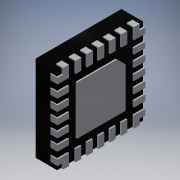
# Autodesk Inventor part: MAX32664GTGA+
Saved by Autodesk Inventor 2018.3 (Build 223284000, 284)
## iProperties
Created: 2021-06-02
Part Number: MAX32664GTGA+
Material: Genérico
Document SubType Name: Modeling
Designer: laguerre
Density: 8.47 g/cm^3
Appearance: Negro
Author: laguerre
Autodesk Inventor part; units mm, degrees
note: some values were not read from the file. Chosen so that the rebuilt part matches the saved one: direction of "Repujado1".
ref_plane "YZ Plane" through (0, 0, 0) normal (1, 0, 0) x (0, 1, 0)
ref_plane "XZ Plane" through (0, 0, 0) normal (0, 1, 0) x (-1, 0, 0)
ref_plane "XY Plane" through (0, 0, 0) normal (0, 0, 1) x (1, 0, 0)
sketch "Boceto39" plane through (0, 0, 0) normal (0, 0, 1) x (1, 0, 0)
  line L0 (-1.5, 1.5) -> (1.5, 1.5)
  line L1 (1.5, 1.5) -> (1.5, -1.5)
  line L2 (1.5, -1.5) -> (-1.5, -1.5)
  line L3 (-1.5, -1.5) -> (-1.5, 1.5)
  point P0 (0, 0)
  point P1 (0, 1.5)
  point P2 (-1.5, 0)
  dimension "d373" = 3
  dimension "d374" = 3
  constraints: 8 end point, 2 midpoint, 2 parallel, 1 horizontal, 1 horizontal alignment, 1 perpendicular, 1 vertical alignment
  measures "d373" distance of L0.start L0.end
  measures "d374" distance of L2.end L0.start
extrude "Extrusión13" add sketch "Boceto39" along normal blind 0.75
sketch "Boceto40" plane through (0, 0, 0.75) normal (0, 0, 1) x (1, 0, 0)
  circle A0 centre (-1.1, 1.1) radius 0.15
  line L0 (-1.5, 1.5) -> (-1.5, -1.5) projected
  line L1 (1.5, 1.5) -> (-1.5, 1.5) projected
  point P0 (0, 0)
  dimension "d377" = 0.4
  dimension "d378" = 0.4
  dimension "d379" = 0.3
  constraints: 1 centre point
  measures "d377" distance from line of L0 A0.centre
  measures "d378" distance from line of A0.centre L1
  measures "d379" diameter of A0
emboss "Repujado1" sketch "Boceto40" operation cut depth 0.001 direction (0, 0, -1)
sketch "Boceto41" plane through (0, 0, 0) normal (0, 0, -1) x (-1, 0, 0)
  line L0 (-0.1, 1.535) -> (0.1, 1.535)
  line L1 (0.1, 1.535) -> (0.1, 1.135)
  line L2 (0.1, 1.135) -> (-0.1, 1.135)
  line L3 (-0.1, 1.135) -> (-0.1, 1.535)
  line L4 (0.3, 1.535) -> (0.5, 1.535)
  line L5 (0.5, 1.535) -> (0.5, 1.135)
  line L6 (0.5, 1.135) -> (0.3, 1.135)
  line L7 (0.3, 1.135) -> (0.3, 1.535)
  line L8 (0.7, 1.535) -> (0.9, 1.535)
  line L9 (0.9, 1.535) -> (0.9, 1.135)
  line L10 (0.9, 1.135) -> (0.7, 1.135)
  line L11 (0.7, 1.135) -> (0.7, 1.535)
  line L12 (-0.5, 1.535) -> (-0.3, 1.535)
  line L13 (-0.3, 1.535) -> (-0.3, 1.135)
  line L14 (-0.3, 1.135) -> (-0.5, 1.135)
  line L15 (-0.5, 1.135) -> (-0.5, 1.535)
  line L16 (-0.9, 1.535) -> (-0.7, 1.535)
  line L17 (-0.7, 1.535) -> (-0.7, 1.135)
  line L18 (-0.7, 1.135) -> (-0.9, 1.135)
  line L19 (-0.9, 1.135) -> (-0.9, 1.535)
  line L20 (-0.1, -1.135) -> (0.1, -1.135)
  line L21 (0.1, -1.135) -> (0.1, -1.535)
  line L22 (0.1, -1.535) -> (-0.1, -1.535)
  line L23 (-0.1, -1.535) -> (-0.1, -1.135)
  line L24 (0.3, -1.135) -> (0.5, -1.135)
  line L25 (0.5, -1.135) -> (0.5, -1.535)
  line L26 (0.5, -1.535) -> (0.3, -1.535)
  line L27 (0.3, -1.535) -> (0.3, -1.135)
  line L28 (0.7, -1.135) -> (0.9, -1.135)
  line L29 (0.9, -1.135) -> (0.9, -1.535)
  line L30 (0.9, -1.535) -> (0.7, -1.535)
  line L31 (0.7, -1.535) -> (0.7, -1.135)
  line L32 (-0.5, -1.135) -> (-0.3, -1.135)
  line L33 (-0.3, -1.135) -> (-0.3, -1.535)
  line L34 (-0.3, -1.535) -> (-0.5, -1.535)
  line L35 (-0.5, -1.535) -> (-0.5, -1.135)
  line L36 (-0.9, -1.135) -> (-0.7, -1.135)
  line L37 (-0.7, -1.135) -> (-0.7, -1.535)
  line L38 (-0.7, -1.535) -> (-0.9, -1.535)
  line L39 (-0.9, -1.535) -> (-0.9, -1.135)
  line L40 (1.135, 0.9) -> (1.535, 0.9)
  line L41 (1.535, 0.9) -> (1.535, 0.7)
  line L42 (1.535, 0.7) -> (1.135, 0.7)
  line L43 (1.135, 0.7) -> (1.135, 0.9)
  line L44 (1.135, 0.5) -> (1.535, 0.5)
  line L45 (1.535, 0.5) -> (1.535, 0.3)
  line L46 (1.535, 0.3) -> (1.135, 0.3)
  line L47 (1.135, 0.3) -> (1.135, 0.5)
  line L48 (1.535, 0.1) -> (1.135, 0.1)
  line L49 (1.135, 0.1) -> (1.135, -0.1)
  line L50 (1.135, -0.1) -> (1.535, -0.1)
  line L51 (1.535, -0.1) -> (1.535, 0.1)
  line L52 (1.135, -0.3) -> (1.535, -0.3)
  line L53 (1.535, -0.3) -> (1.535, -0.5)
  line L54 (1.535, -0.5) -> (1.135, -0.5)
  line L55 (1.135, -0.5) -> (1.135, -0.3)
  line L56 (1.535, -0.7) -> (1.135, -0.7)
  line L57 (1.135, -0.7) -> (1.135, -0.9)
  line L58 (1.135, -0.9) -> (1.535, -0.9)
  line L59 (1.535, -0.9) -> (1.535, -0.7)
  line L60 (-1.535, 0.9) -> (-1.135, 0.9)
  line L61 (-1.135, 0.9) -> (-1.135, 0.7)
  line L62 (-1.135, 0.7) -> (-1.535, 0.7)
  line L63 (-1.535, 0.7) -> (-1.535, 0.9)
  line L64 (-1.535, 0.5) -> (-1.135, 0.5)
  line L65 (-1.135, 0.5) -> (-1.135, 0.3)
  line L66 (-1.135, 0.3) -> (-1.535, 0.3)
  line L67 (-1.535, 0.3) -> (-1.535, 0.5)
  line L68 (-1.135, 0.1) -> (-1.535, 0.1)
  line L69 (-1.535, 0.1) -> (-1.535, -0.1)
  line L70 (-1.535, -0.1) -> (-1.135, -0.1)
  line L71 (-1.135, -0.1) -> (-1.135, 0.1)
  line L72 (-1.535, -0.3) -> (-1.135, -0.3)
  line L73 (-1.135, -0.3) -> (-1.135, -0.5)
  line L74 (-1.135, -0.5) -> (-1.535, -0.5)
  line L75 (-1.535, -0.5) -> (-1.535, -0.3)
  line L76 (-1.135, -0.7) -> (-1.535, -0.7)
  line L77 (-1.535, -0.7) -> (-1.535, -0.9)
  line L78 (-1.535, -0.9) -> (-1.135, -0.9)
  line L79 (-1.135, -0.9) -> (-1.135, -0.7)
  line L80 (1.5, 1.5) -> (-1.5, 1.5) projected
  line L81 (1.5, -1.5) -> (1.5, 1.5) projected
  line L82 (-1.5, 1.5) -> (-1.5, -1.5) projected
  line L83 (-1.5, -1.5) -> (1.5, -1.5) projected
  line L84 (1.135, 1.535) -> (1.135, 1.135)
  line L85 (1.135, 1.135) -> (1.535, 1.135)
  line L86 (1.535, 1.135) -> (1.535, 1.335)
  line L87 (1.535, 1.335) -> (1.335, 1.335)
  line L88 (1.335, 1.335) -> (1.335, 1.535)
  line L89 (-1.5, 1.5) -> (1.5, 1.5) projected
  line L90 (1.335, 1.535) -> (1.135, 1.535)
  line L91 (-1.135, 1.535) -> (-1.135, 1.135)
  line L92 (-1.135, 1.135) -> (-1.535, 1.135)
  line L93 (-1.535, 1.135) -> (-1.535, 1.335)
  line L94 (-1.535, 1.335) -> (-1.335, 1.335)
  line L95 (-1.335, 1.335) -> (-1.335, 1.535)
  line L96 (-1.335, 1.535) -> (-1.135, 1.535)
  line L97 (1.135, -1.135) -> (1.135, -1.535)
  line L98 (1.135, -1.535) -> (1.335, -1.535)
  line L99 (1.335, -1.535) -> (1.335, -1.335)
  line L100 (1.335, -1.335) -> (1.535, -1.335)
  line L101 (1.535, -1.335) -> (1.535, -1.135)
  line L102 (1.535, -1.135) -> (1.135, -1.135)
  line L103 (-1.535, -1.135) -> (-1.135, -1.135)
  line L104 (-1.135, -1.135) -> (-1.135, -1.535)
  line L105 (-1.135, -1.535) -> (-1.335, -1.535)
  line L106 (-1.335, -1.535) -> (-1.335, -1.335)
  line L107 (-1.335, -1.335) -> (-1.535, -1.335)
  line L108 (-1.535, -1.335) -> (-1.535, -1.135)
  line L109 (-0.85, 0.85) -> (0.55, 0.85)
  line L110 (0.85, 0.55) -> (0.85, -0.85)
  line L111 (0.85, -0.85) -> (-0.85, -0.85)
  line L112 (-0.85, -0.85) -> (-0.85, 0.85)
  line L113 (0.55, 0.85) -> (0.85, 0.55)
  point P0 (0, 0)
  point P1 (0, -1.135)
  point P2 (0, 1.135)
  point P3 (0.4, -1.135)
  point P4 (0.4, 1.135)
  point P5 (0.8, 1.135)
  point P6 (0.8, -1.135)
  point P7 (-0.4, -1.135)
  point P8 (-0.4, 1.135)
  point P9 (-0.8, -1.135)
  point P10 (-0.8, 1.135)
  point P11 (1.135, 0)
  point P12 (-1.535, 0)
  point P13 (-1.135, 0.8)
  point P14 (1.135, 0.8)
  point P15 (1.135, 0.4)
  point P16 (-1.135, 0.4)
  point P17 (-1.135, 0)
  point P18 (-1.135, -0.4)
  point P19 (1.135, -0.4)
  point P20 (1.135, -0.8)
  point P21 (-1.135, -0.8)
  point P22 (0.85, 0.85)
  point P23 (-0.85, 0)
  point P24 (0, -0.85)
  dimension "d382" = 0.2
  dimension "d384" = 0.4
  dimension "d385" = 0.2
  dimension "d386" = 0.4
  dimension "d387" = 0.4
  dimension "d388" = 0.4
  dimension "d389" = 0.4
  dimension "d390" = 0.4
  dimension "d391" = 0.4
  dimension "d392" = 0.4
  dimension "d393" = 0.4
  dimension "d394" = 0.4
  dimension "d396" = 0.035
  dimension "d397" = 0.035
  dimension "d398" = 0.035
  dimension "d399" = 0.035
  dimension "d400" = 0.3
  dimension "d401" = 0.3
  dimension "d402" = 1.7
  constraints: 218 end point, 42 parallel, 39 equal length, 39 perpendicular, 23 midpoint, 22 horizontal, 20 collinear, 20 point on line, 7 horizontal alignment, 7 vertical alignment, 3 vertical
  measures "d382" distance of L0.start L0.end
  measures "d384" distance of L2.end L0.start
  measures "d385" distance of L20.start L20.end
  measures "d386" distance of L22.end L20.start
  measures "d387" distance of point (0.4, -1.135) point (0, -1.135)
  measures "d388" distance of point (0.8, -1.135) point (0.4, -1.135)
  measures "d389" distance of point (0, -1.135) point (-0.4, -1.135)
  measures "d390" distance of point (-0.4, -1.135) point (-0.8, -1.135)
  measures "d391" distance of point (-1.135, 0.8) point (-1.135, 0.4)
  measures "d392" distance of point (-1.135, 0.4) point (-1.135, 0)
  measures "d393" distance of point (-1.135, -0.4) point (-1.135, 0)
  measures "d394" distance of point (-1.135, -0.4) point (-1.135, -0.8)
  measures "d396" distance between parallel lines of L8 L80
  measures "d397" distance between parallel lines of L81 L41
  measures "d398" distance between parallel lines of L82 L63
  measures "d399" distance between parallel lines of L83 L30
  measures "d400" distance of L109.end point (0.85, 0.85)
  measures "d401" distance of L110.start point (0.85, 0.85)
  measures "d402" distance between parallel lines of L110 L112
extrude "Extrusión14" add sketch "Boceto41" along normal blind 0.05 and the other way blind 0.203 contours L0 L1 L80 L3 | L80 L1 L2 L3 | L80 L15 L12 L13 | L13 L14 L15 L80 | L80 L5 L6 L7 | L7 L4 L5 L80 | L80 L19 L16 L17 | L17 L18 L19 L80 | L80 L9 L10 L11 | L11 L8 L9 L80 | L91 L92 L82 L94 L95 L80 | L80 L95 L96 L91 | L84 L90 L88 L80 | L80 L88 L87 L81 L85 L84 | L92 L93 L94 L82 | L81 L87 L86 L85 | L82 L62 L63 L60 | L60 L61 L62 L82 | L81 L42 L43 L40 | L40 L41 L42 L81 | L82 L66 L67 L64 | L64 L65 L66 L82 | L81 L46 L47 L44 | L44 L45 L46 L81 | L82 L70 L69 L68 | L68 L71 L70 L82 | L81 L50 L49 L48 | L48 L51 L50 L81 | L82 L74 L75 L72 | L72 L73 L74 L82 | L81 L54 L55 L52 | L52 L53 L54 L81 | L82 L78 L77 L76 | L76 L79 L78 L82 | L81 L58 L57 L56 | L56 L59 L58 L81 | L103 L104 L83 L106 L107 L82 | L82 L107 L108 L103 | L102 L101 L100 L81 | L81 L100 L99 L83 L97 L102 | L104 L105 L106 L83 | L83 L99 L98 L97 | L83 L37 L38 L39 | L39 L36 L37 L83 | L83 L31 L28 L29 | L29 L30 L31 L83 | L83 L33 L34 L35 | L35 L32 L33 L83 | L83 L27 L24 L25 | L25 L26 L27 L83 | L83 L21 L22 L23 | L23 L20 L21 L83 | L109 L113 L110 L111 L112
